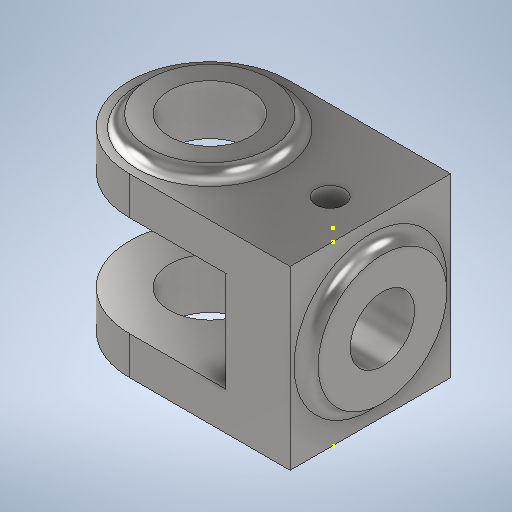
# Autodesk Inventor part: nakrętka
Saved by Autodesk Inventor 2025.2 (Build 292293000, 293)
## iProperties
Created: 2025-03-16
Part Number: nakrętka
Material: Stal nierdzewna, austenityczna
Document SubType Name: Modeling
Designer: barte
Density: 8 g/cm^3
Appearance: Częściowo polerowany
Author: barte
Autodesk Inventor part; units mm, degrees
ref_plane "YZ Plane" through (0, 0, 0) normal (1, 0, 0) x (0, 1, 0)
ref_plane "XZ Plane" through (0, 0, 0) normal (0, 1, 0) x (-1, 0, 0)
ref_plane "XY Plane" through (0, 0, 0) normal (0, 0, 1) x (1, 0, 0)
sketch "Szkic1" plane through (0, 0, 0) normal (0, 1, 0) x (-1, 0, 0)
  line L0 (0, 10.6544) -> (0, -29.3456)
  line L1 (0, -29.3456) -> (40, -29.3456)
  line L2 (0, 10.6544) -> (40, 10.6544)
  arc A0 (40, -29.3456) -> (40, 10.6544) centre (40, -9.3456) ccw
  point P0 (0, 0)
  dimension "d0" = 40
  dimension "d1" = 40
  constraints: 6 end point, 2 point on circle, 1 centre point, 1 horizontal, 1 perpendicular, 1 tangent, 1 vertical
  measures "d0" distance of L0.start L0.end
  measures "d1" distance of L0.end L1.end
extrude "Wyciągnięcie proste1" add sketch "Szkic1" along normal blind 9.5
sketch "Szkic2" plane through (0, 9.5, 0) normal (0, 1, 0) x (1, 0, 0)
  line L0 (-40, -10.6544) -> (0, -10.6544) projected
  line L1 (0.0007, -10.6544) -> (-40, -10.6544)
  arc A0 (-40, 29.3456) -> (-40, -10.6544) centre (-40, 9.3456) ccw projected
  circle A1 centre (-40, 9.3456) radius 15
  circle A2 centre (-40, 9.3456) radius 10
  point P0 (0, 0)
  dimension "d4" = 30
  dimension "d5" = 20
  constraints: 3 coincident, 2 centre point, 2 end point, 1 horizontal
  measures "d4" diameter of A1
  measures "d5" diameter of A2
extrude "Wyciągnięcie proste2" add sketch "Szkic2" along normal blind 3
fillet "Zaokrąglenie1" radius 3 1 edges at (-55, 9.5, -9.3456)
sketch "Szkic3" plane through (0, 0, 0) normal (0, -1, 0) x (1, 0, 0)
  line L0 (0, 10.6544) -> (0, -29.3456) projected
  line L1 (0, -29.3456) -> (-16, -29.3456)
  line L2 (0, -29.3456) -> (-40, -29.3456) projected
  line L3 (-16, -29.3456) -> (-16, 10.6544)
  line L4 (-40, 10.6544) -> (0, 10.6544) projected
  line L5 (-16, 10.6544) -> (0, 10.6544)
  line L6 (0, 10.6544) -> (0, -29.3456)
  point P0 (0, 0)
  dimension "d9" = 16
  dimension "d10" = 40
  constraints: 8 end point, 2 collinear, 2 point on line
  measures "d9" distance of L0.end L1.end
  measures "d10" distance of L1.end L3.end
extrude "Wyciągnięcie proste3" add sketch "Szkic3" along normal blind 12.5
sketch "Szkic4" plane through (-40, 9.5, -9.3456) normal (0, 1, 0) x (1, 0, 0)
  point P0 (40, -9.3456)
mirror "Odbij1" about plane through (-8, -12.5, -9.3456) normal (0, -1, 0)
sketch "Szkic7" plane through (0, 9.5, 10.6544) normal (1, 0, 0) x (0, 0, -1)
  point P0 (10.6544, -9.5)
sketch "Szkic8" plane through (0, 9.5, 10.6544) normal (1, 0, 0) x (0, 0, -1)
  point P0 (10.6544, -9.5)
sketch "Szkic9" plane through (0, 9.5, 10.6544) normal (1, 0, 0) x (0, 0, -1)
  line L0 (40, 0) -> (0, 0) projected
  line L1 (0, 0) -> (0, -22)
  line L2 (0, -44) -> (0, 0) projected
  line L3 (0, -22) -> (20, -22)
  circle A0 centre (20, -22) radius 16
  circle A1 centre (20, -22) radius 8
  point P0 (10.6544, -9.5)
  dimension "d15" = 22
  dimension "d16" = 32
  dimension "d17" = 16
  constraints: 4 end point, 2 centre point, 2 coincident, 1 midpoint
  measures "d15" distance of L0.end L1.end
  measures "d16" diameter of A0
  measures "d17" diameter of A1
extrude "Wyciągnięcie proste4" cut sketch "Szkic9" against normal blind 20 contours A1
sketch "Szkic10" plane through (0, 9.5, 10.6544) normal (1, 0, 0) x (0, 0, -1)
  line L0 (0, -9.5) -> (0, 0) projected
  line L1 (0, 0) -> (0, -22)
  line L2 (0, -22) -> (20, -22)
  circle A0 centre (20, -22) radius 16
  point P0 (10.6544, -9.5)
  dimension "d20" = 22
  dimension "d21" = 20
  dimension "d22" = 32
  constraints: 4 end point, 1 centre point, 1 coincident, 1 collinear, 1 perpendicular
  measures "d20" distance of L0.end L1.end
  measures "d21" distance of L1.end L2.end
  measures "d22" diameter of A0
extrude "Wyciągnięcie proste5" add sketch "Szkic10" along normal blind 3
fillet "Zaokrąglenie2" radius 3 1 edges at (0, -12.5, 6.6544)
sketch "Szkic11" plane through (3, -12.5, -9.3456) normal (1, 0, 0) x (0, 0, -1)
  circle A0 centre (0, 0) radius 8
  point P0 (-9.3456, 12.5)
  dimension "d26" = 16
  constraints: 1 centre point
  measures "d26" diameter of A0
extrude "Wyciągnięcie proste6" cut sketch "Szkic11" against normal blind 20
sketch "Szkic12" plane through (0, 0, 0) normal (0, -1, 0) x (1, 0, 0)
  point P0 (0, 0)
sketch "Szkic13" plane through (-40, -34.5, -9.3456) normal (0, -1, 0) x (1, 0, 0)
  point P0 (40, 9.3456)
sketch "Szkic14" plane through (-40, 12.5, -9.3456) normal (0, 1, 0) x (1, 0, 0)
  point P0 (40, -9.3456)
sketch "Szkic15" plane through (-40, 9.5, -9.3456) normal (0, 1, 0) x (1, 0, 0)
  circle A0 centre (0, 0) radius 10
  point P0 (40, -9.3456)
  dimension "d29" = 20
  constraints: 1 centre point
  measures "d29" diameter of A0
extrude "Wyciągnięcie proste7" cut sketch "Szkic15" against normal blind 9.5
sketch "Szkic16" plane through (-40, -34.5, -9.3456) normal (0, -1, 0) x (1, 0, 0)
  circle A0 centre (0, 0) radius 10
  point P0 (40, 9.3456)
  dimension "d32" = 20
  constraints: 1 centre point
  measures "d32" diameter of A0
extrude "Wyciągnięcie proste8" cut sketch "Szkic16" against normal blind 9.5
sketch "Szkic17" plane through (0, 9.5, 0) normal (0, 1, 0) x (1, 0, 0)
  line L0 (0, -10.6544) -> (0, 29.3456) projected
  line L1 (0, 9.3456) -> (-10, 9.3456)
  point P0 (0, 0)
  constraints: 2 end point, 1 horizontal, 1 midpoint
hole "Otwór1" at (-10, 9.5, -9.3456) direction (0, -1, 0) diameter 7 depth 75.75 tip angle 118
